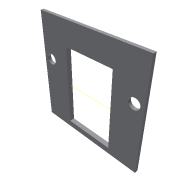
# Autodesk Inventor part: 20_Cube_Insert_Beamsplittercube_Dichroicmirror_Retainplate
Saved by Autodesk Inventor 2019 (Build 230136000, 136)
## iProperties
Created: 2019-08-12
Part Number: 20_Cube_Insert_Beamsplittercube_Dichroicmirror_Retainplate
Material: Generic
Document SubType Name: Modeling
Designer: diederichbenedict
Density: 1 g/cm^3
Appearance: Default
Author: diederichbenedict
Autodesk Inventor part; units mm, degrees
ref_plane "YZ Plane" through (0, 0, 0) normal (1, 0, 0) x (0, 1, 0)
ref_plane "XZ Plane" through (0, 0, 0) normal (0, 1, 0) x (-1, 0, 0)
ref_plane "XY Plane" through (0, 0, 0) normal (0, 0, 1) x (1, 0, 0)
ref_plane "Work Plane1" through (0, 0, 0) normal (0, 0, 1) x (1, 0, 0)
sketch "Sketch1" plane through (0, 0, 0) normal (0, 0, 1) x (1, 0, 0)
  line L0 (-8.5, -13) -> (-8.5, 13) construction
  line L1 (-8.5, 13) -> (8.5, 13) construction
  line L2 (8.5, 13) -> (8.5, -13) construction
  line L3 (8.5, -13) -> (-8.5, -13) construction
  line L4 (-11.5, -16) -> (11.5, -16) construction
  line L5 (11.5, -16) -> (11.5, 16) construction
  line L6 (11.5, 16) -> (-11.5, 16) construction
  line L7 (-11.5, 16) -> (-11.5, -16) construction
  circle A0 centre (13.8009, 6.2056) radius 1.4 construction
  circle A1 centre (-13.8009, 6.2056) radius 1.4 construction
  line L8 (16.5, -19) -> (-16.5, -19)
  line L9 (-16.5, -19) -> (-16.5, 19)
  line L10 (-16.5, 19) -> (16.5, 19)
  line L11 (16.5, 19) -> (16.5, -19)
  line L12 (16.5, -19) -> (-16.5, 19) construction
  line L13 (-16.5, -19) -> (16.5, 19) construction
  circle A2 centre (-13.8009, 6.2056) radius 1.6
  circle A3 centre (13.8009, 6.2056) radius 1.6
  line L14 (-7.5, 12) -> (7.5, 12)
  line L15 (7.5, 12) -> (7.5, -12)
  line L16 (7.5, -12) -> (-7.5, -12)
  line L17 (-7.5, -12) -> (-7.5, 12)
  line L18 (-7.5, 12) -> (7.5, -12) construction
  line L19 (7.5, 12) -> (-7.5, -12) construction
  line L20 (16.5, -14) -> (-16.5, -14)
  point P0 (0, 0)
  dimension "d0" = 33
  dimension "d1" = 38
  dimension "d2" = 3.2
  dimension "d3" = 3.2
  dimension "d4" = 15
  dimension "d5" = 24
  dimension "d11" = 5
  constraints: 26 end point, 4 midpoint, 4 parallel, 3 perpendicular, 2 centre point, 2 coincident, 2 horizontal, 2 point on line
  measures "d0" distance of L9.end L10.end
  measures "d1" distance of L8.end L9.end
  measures "d2" diameter of A2
  measures "d3" diameter of A3
  measures "d4" distance of L15.end L16.end
  measures "d5" distance of L14.end L15.end
  measures "d11" distance between parallel lines of L20 L8
extrude "Extrusion1" add sketch "Sketch1" along normal blind 1 contours L20 L9 L10 L11
sketch "Sketch2" plane through (0, 0, 0) normal (0, 0, -1) x (-1, 0, 0)
  line L0 (-7.5, -12) -> (-7.5, 12) projected
  line L1 (-7.5, 12) -> (7.5, 12) projected
  line L2 (7.5, 12) -> (7.5, -12) projected
  line L3 (7.5, -12) -> (-7.5, -12) projected
  circle A0 centre (-13.8009, 6.2056) radius 1.6 projected
  circle A1 centre (13.8009, 6.2056) radius 1.6 projected
  line L4 (16.5, 19) -> (16.5, -14) projected
  line L5 (-16.5, 19) -> (16.5, 19) projected
  line L6 (-16.5, -14) -> (-16.5, 19) projected
  line L7 (8.5, -13) -> (8.5, 13)
  line L8 (8.5, 13) -> (-8.5, 13)
  line L9 (-8.5, 13) -> (-8.5, -13)
  line L10 (-8.5, -13) -> (8.5, -13)
  line L11 (16.5, -14) -> (-16.5, -14) projected
  point P0 (0, 0)
  dimension "d8" = 1
  constraints: 8 end point, 3 other
  measures "d8" distance between parallel lines of L2 L7
extrude "Extrusion2" add sketch "Sketch2" along normal blind 0.5 contours L10 L9 L8 L7
body "Solid1"
